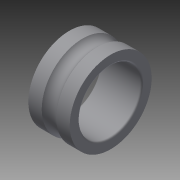
# Autodesk Inventor part: WBC6-12ZZ Inner ring
Saved by Autodesk Inventor 2014 SP2 (Build 180246200, 246)
## iProperties
Created: 2019-09-21
Part Number: WBC6-12ZZ Inner ring
Material: Generic
Catalog Web Link: www.cadenas.de
Description: Six types ir-Metric system sizes
Vendor: NTN
Document SubType Name: Modeling
Designer: psadmin
Manufacturer: NTN
Mass: 0.0755622 g
Surface Area: 2.17606 cm^2
Volume: 0.0755622 cm^3
Density: 1 g/cm^3
Appearance: PSOLRGB-192-192-192
Category: PARTsolutions
Company: NTN
Title: WBC6-12ZZ Inner ring
Author: Cadenas PARTsolutions
Comments: Metric system sizes
PSOL_IDENT_0: {$CADENAS_DATA\23d-libs\ntn\ball_roller_bearings\miniature_extra_small_bb\metric_system_sizes\mss_ir
PSOL_IDENT_1: .prj},189 {VTYP=3D},{NB=WBC6-12ZZ Inner ring},{LINA=WBC6-12ZZ Inner ring},{NN=Six types ir},{DATE=29
PSOL_IDENT_2: .01.2019 23:03:31},{GEOMDATE=28.06.2007 12:57:00},{VERSION=},{LINEID=12850},{WBVAR=},{WBNUMERIC=}  {
PSOL_IDENT_3: NB=WBC6-12ZZ Inner ring},{LINA=WBC6-12ZZ Inner ring},{KT=DUMMY},{IDNR=},{SD=6.0},{D=12},{B=3.0},{R=0
PSOL_IDENT_4: .15},{ORDER=WBC6-12ZZ},{CR=830},{COR=365},{CRF=85},{CORF=37},{LSG=40 000},{LSO=47 000},{MASS=1.30},{
PSOL_IDENT_5: D1=13.2},{D2=13.6},{C1=0.6},{C2=0.8},{ORDER1=BC6-12},{WSS=WBC6-12ZZ},{WDS=ZZ},{UTWF=FLBC6-12},{FORSS=
PSOL_IDENT_6: FLAWBC6-12Z},{FORDS=ZZ},{DA1=7,2},{DA2=7,9},{DA=10,8},{RAS=0,15},{MASS1=1.40},{B1=4.0},{VERS=3},{X=3
PSOL_IDENT_7: },{N=9},{O=28.26},{RB=0.888}
NN: Six types ir
NT: Metric system sizes
NB: WBC6-12ZZ Inner ring
NBSYN: $ORDER. Inner ring
LINA: WBC6-12ZZ Inner ring
SD: 6
D: 12
B: 3
R: 0.15
CR: 830
COR: 365
CRF: 85
CORF: 37
LSG: 40 000
LSO: 47 000
MASS: 1.3
D1: 13.2
D2: 13.6
C1: 0.6
C2: 0.8
ORDER1: BC6-12
WSS: WBC6-12ZZ
WDS: ZZ
UTWF: FLBC6-12
FORSS: FLAWBC6-12Z
FORDS: ZZ
DA1: 7,2
DA2: 7,9
DA: 10,8
RAS: 0,15
MASS1: 1.4
B1: 4
VERS: 3
SUPPLIER: NTN
ARTICLENO: WBC6-12ZZ Inner ring
BOMINFO: WBC6-12ZZ Inner ring
CREATOR: CADENAS GmbH
Autodesk Inventor part; units mm, degrees
sketch "Sketch_2" plane through (0, 0, 0) normal (0, 0, 1) x (1, 0, 0)
  line L0 (4, 0) -> (0, 0)
  arc A0 (0, 3.15) -> (0.15, 3) centre (0.15, 3.15) ccw
  line L1 (0.15, 3) -> (3.85, 3)
  arc A1 (3.85, 3) -> (4, 3.15) centre (3.85, 3.15) ccw
  line L2 (4, 3.15) -> (4, 3.96)
  line L3 (4, 3.96) -> (2.7049, 3.96)
  arc A2 (1.2951, 3.96) -> (2.7049, 3.96) centre (2, 4.5) ccw
  line L4 (1.2951, 3.96) -> (0, 3.96)
  line L5 (0, 3.96) -> (0, 3.15)
  constraints: 12 end point, 6 point on circle, 3 centre point
revolve "Revolution1" add sketch "Sketch_2" angle 360 about axis through (4, 0, 0) along (1, 0, 0)
ref_plane "mss_ir_XY" through (0, 0, 0) normal (1, 0, 0) x (0, 0, -1)
ref_plane "mss_ir_YZ" through (0, 0, 0) normal (0, 0, -1) x (0, 1, 0)
ref_plane "mss_ir_ZX" through (0, 0, 0) normal (0, 1, 0) x (1, 0, 0)
body "Solid1"
